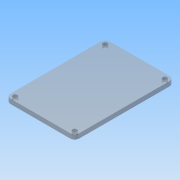
# Autodesk Inventor part: ET-40_Cover
Saved by Autodesk Inventor 2014 SP2 (Build 180246200, 246)
## iProperties
Created: 2015-05-11
Part Number: ET-40_Cover
Material: ポリカーボネート、クリア
Document SubType Name: Modeling
Designer: andou
Density: 1.2 g/cm^3
Appearance: ポリカーボネート - クリア
Author: andou
Autodesk Inventor part; units mm, degrees
ref_plane "YZ Plane" through (0, 0, 0) normal (1, 0, 0) x (0, 1, 0)
ref_plane "XZ Plane" through (0, 0, 0) normal (0, 1, 0) x (-1, 0, 0)
ref_plane "XY Plane" through (0, 0, 0) normal (0, 0, 1) x (1, 0, 0)
sketch "スケッチ1" plane through (0, 0, 0) normal (0, 0, 1) x (1, 0, 0)
  line L0 (19.5, -32.5) -> (-19.5, -32.5)
  line L1 (-22.5, -29.5) -> (-22.5, 29.5)
  line L2 (-19.5, 32.5) -> (19.5, 32.5)
  line L3 (22.5, 29.5) -> (22.5, -29.5)
  line L4 (22.5, -32.5) -> (-22.5, 32.5) construction
  line L5 (-22.5, -32.5) -> (22.5, 32.5) construction
  arc A0 (-19.5, 32.5) -> (-22.5, 29.5) centre (-19.5, 29.5) ccw
  arc A1 (22.5, 29.5) -> (19.5, 32.5) centre (19.5, 29.5) ccw
  arc A2 (19.5, -32.5) -> (22.5, -29.5) centre (19.5, -29.5) ccw
  arc A3 (-22.5, -29.5) -> (-19.5, -32.5) centre (-19.5, -29.5) ccw
  point P0 (0, 0)
  dimension "d0" = 45
  dimension "d1" = 65
  dimension "d2" = 3
  constraints: 12 end point, 8 point on circle, 8 point on line, 8 tangent, 4 centre point, 3 equal radius, 2 midpoint, 2 parallel, 1 horizontal, 1 perpendicular
  measures "d0" distance of L4.start L5.start
  measures "d1" distance of L5.start L4.end
  measures "d2" radius of A0
extrude "押し出し1" add sketch "スケッチ1" along normal blind 3
sketch "スケッチ2" plane through (0, 0, 3) normal (0, 0, 1) x (1, 0, 0)
  arc A0 (-19.5, 32.5) -> (-22.5, 29.5) centre (-19.5, 29.5) ccw projected
  arc A1 (-22.5, -29.5) -> (-19.5, -32.5) centre (-19.5, -29.5) ccw projected
  arc A2 (19.5, -32.5) -> (22.5, -29.5) centre (19.5, -29.5) ccw projected
  arc A3 (22.5, 29.5) -> (19.5, 32.5) centre (19.5, 29.5) ccw projected
  circle A4 centre (-19.5, 29.5) radius 1.5
  circle A5 centre (19.5, 29.5) radius 1.5
  circle A6 centre (19.5, -29.5) radius 1.5
  circle A7 centre (-19.5, -29.5) radius 1.5
  point P0 (0, 0)
  dimension "d5" = 3
  constraints: 4 centre point, 4 coincident, 3 equal radius
  measures "d5" diameter of A4
hole "穴1" at (-19.5, -29.5, 3) at (19.5, -29.5, 3) at (19.5, 29.5, 3) at (-19.5, 29.5, 3) direction (0, 0, -1) diameter 3 end through all
